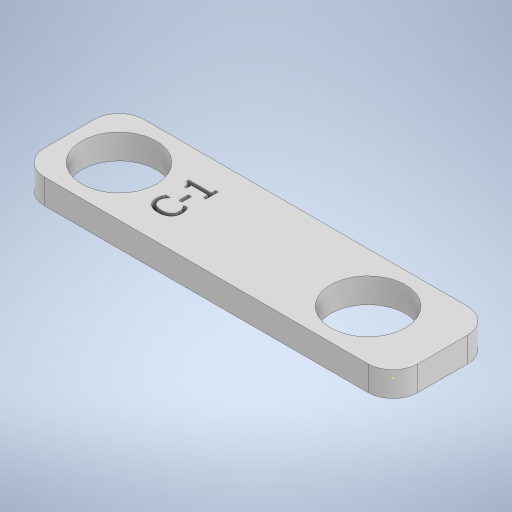
# Autodesk Inventor part: Parts_Combiner
Saved by Autodesk Inventor 2024.3 (Build 283343000, 343)
## iProperties
Created: 2024-08-06
Part Number: Parts_Combiner
Material: Generic
Document SubType Name: Modeling
Designer: lordk
Density: 1 g/cm^3
Appearance: Default
Author: lordk
Autodesk Inventor part; units mm, degrees
ref_plane "YZ Plane" through (0, 0, 0) normal (1, 0, 0) x (0, 1, 0)
ref_plane "XZ Plane" through (0, 0, 0) normal (0, 1, 0) x (-1, 0, 0)
ref_plane "XY Plane" through (0, 0, 0) normal (0, 0, 1) x (1, 0, 0)
sketch "Sketch1" plane through (0, 0, 0) normal (0, 1, 0) x (-1, 0, 0)
  line L0 (0, 0) -> (15, 0)
  line L1 (15, 0) -> (15, -4)
  line L2 (15, -4) -> (0, -4)
  line L3 (0, -4) -> (0, 0)
  dimension "d0" = 15
  dimension "d1" = 4
  constraints: 8 end point, 2 parallel, 1 horizontal, 1 perpendicular
  measures "d0" distance of L1.end L2.end
  measures "d1" distance of L0.end L1.end
extrude "Extrusion1" add sketch "Sketch1" along normal blind 1
sketch "Sketch2" plane through (0, 1, 0) normal (0, 1, 0) x (1, 0, 0)
  line L0 (0, 4) -> (-15, 4) projected
  line L1 (-15, 4) -> (-15, 0) projected
  point P0 (0, 0)
  point P1 (-13, 2)
  dimension "d18" = 2
  dimension "d19" = 2
  measures "d18" distance from line of L0 point (-13, 2)
  measures "d19" distance from line of L1 point (-13, 2)
hole "Hole1" at (-13, 1, -2) direction (0, -1, 0) diameter 3 depth 5 tip angle 118
sketch "Sketch3" plane through (0, 1, 0) normal (0, 1, 0) x (1, 0, 0)
  line L0 (0, 0) -> (0, 4) projected
  line L1 (0, 4) -> (-15, 4) projected
  point P0 (-3, 2)
  dimension "d20" = 3
  dimension "d21" = 2
  measures "d20" distance from line of L0 point (-3, 2)
  measures "d21" distance from line of L1 point (-3, 2)
hole "Hole2" at (-3, 1, -2) direction (0, -1, 0) diameter 3 depth 5 tip angle 118
sketch "Sketch4" plane through (0, 1, 0) normal (0, 1, 0) x (1, 0, 0)
  point P0 (0, 0)
fillet "Fillet1" radius 1 4 edges at (0, 0.5, 0) (0, 0.5, -4) (-15, 0.5, 0) (-15, 0.5, -4)
sketch "Sketch5" plane through (0, 1, 0) normal (0, 1, 0) x (1, 0, 0)
  line L0 (-11, 1) -> (-11, 3) construction
  line L1 (-11, 3) -> (-5, 3) construction
  line L2 (-5, 3) -> (-5, 1) construction
  line L3 (-5, 1) -> (-11, 1) construction
  line L4 (-1, 4) -> (-14, 4) projected
  line L5 (-14, 0) -> (-1, 0) projected
  line L6 (0, 1) -> (0, 3) projected
  line L7 (-15, 3) -> (-15, 1) projected
  spline S0 degree 2 poles (-9.9643, 1.4919) (-9.9643, 1.3947) (-10.03, 1.2301) (-10.0956, 1.1702) knots 0 0 0 1 2 2 2
  spline S1 degree 2 poles (-10.0956, 1.1702) (-10.1605, 1.1102) (-10.3549, 1.0446) (-10.4814, 1.0446) knots 0 0 0 1 2 2 2
  spline S2 degree 2 poles (-10.4814, 1.0446) (-10.607, 1.0446) (-10.7934, 1.1086) (-10.8622, 1.1694) knots 0 0 0 1 2 2 2
  spline S3 degree 2 poles (-10.8622, 1.1694) (-10.9295, 1.2293) (-11, 1.393) (-11, 1.4943) knots 0 0 0 1 2 2 2
  spline S4 degree 2 poles (-11, 1.4943) (-11, 1.5446) (-10.9854, 1.6329) (-10.9741, 1.6702) knots 0 0 0 1 2 2 2
  spline S5 degree 2 poles (-10.9741, 1.6702) (-10.9635, 1.7026) (-10.9335, 1.7699) (-10.9157, 1.8031) knots 0 0 0 1 2 2 2
  line L8 (-10.9157, 1.8031) -> (-10.7553, 1.8031)
  line L9 (-10.7553, 1.8031) -> (-10.7553, 1.7925)
  spline S6 degree 2 poles (-10.7553, 1.7925) (-10.7715, 1.7747) (-10.8169, 1.7196) (-10.8387, 1.6799) knots 0 0 0 1 2 2 2
  spline S7 degree 2 poles (-10.8387, 1.6799) (-10.8598, 1.6418) (-10.8865, 1.5519) (-10.8865, 1.4935) knots 0 0 0 1 2 2 2
  spline S8 degree 2 poles (-10.8865, 1.4935) (-10.8865, 1.4295) (-10.8339, 1.3152) (-10.7836, 1.2723) knots 0 0 0 1 2 2 2
  spline S9 degree 2 poles (-10.7836, 1.2723) (-10.7326, 1.2301) (-10.5778, 1.1831) (-10.4814, 1.1831) knots 0 0 0 1 2 2 2
  spline S10 degree 2 poles (-10.4814, 1.1831) (-10.3784, 1.1831) (-10.2301, 1.2326) (-10.1791, 1.2755) knots 0 0 0 1 2 2 2
  spline S11 degree 2 poles (-10.1791, 1.2755) (-10.1297, 1.3177) (-10.0794, 1.4303) (-10.0794, 1.4935) knots 0 0 0 1 2 2 2
  spline S12 degree 2 poles (-10.0794, 1.4935) (-10.0794, 1.5511) (-10.1078, 1.6491) (-10.1288, 1.6872) knots 0 0 0 1 2 2 2
  spline S13 degree 2 poles (-10.1288, 1.6872) (-10.1499, 1.7237) (-10.1937, 1.778) (-10.2091, 1.7934) knots 0 0 0 1 2 2 2
  line L10 (-10.2091, 1.7934) -> (-10.2091, 1.8031)
  line L11 (-10.2091, 1.8031) -> (-10.0502, 1.8031)
  spline S14 degree 2 poles (-10.0502, 1.8031) (-10.0348, 1.7699) (-10.0065, 1.7115) (-9.9935, 1.6702) knots 0 0 0 1 2 2 2
  spline S15 degree 2 poles (-9.9935, 1.6702) (-9.9789, 1.6264) (-9.9643, 1.5519) (-9.9643, 1.4919) knots 0 0 0 1 2 2 2
  line L12 (-10.359, 2.265) -> (-10.359, 1.8865)
  line L13 (-10.359, 1.8865) -> (-10.4806, 1.8865)
  line L14 (-10.4806, 1.8865) -> (-10.4806, 2.265)
  line L15 (-10.4806, 2.265) -> (-10.359, 2.265)
  line L16 (-9.9822, 2.9643) -> (-9.9822, 2.4765)
  line L17 (-9.9822, 2.4765) -> (-10.0843, 2.4765)
  line L18 (-10.0843, 2.4765) -> (-10.0843, 2.658)
  line L19 (-10.0843, 2.658) -> (-10.7545, 2.658)
  line L20 (-10.7545, 2.658) -> (-10.7545, 2.4765)
  line L21 (-10.7545, 2.4765) -> (-10.846, 2.4765)
  spline S16 degree 2 poles (-10.846, 2.4765) (-10.846, 2.5794) (-10.9044, 2.6767) (-10.9854, 2.6831) knots 0 0 0 1 2 2 2
  line L22 (-10.9854, 2.6831) -> (-10.9854, 2.7869)
  line L23 (-10.9854, 2.7869) -> (-10.0843, 2.7869)
  line L24 (-10.0843, 2.7869) -> (-10.0843, 2.9643)
  line L25 (-10.0843, 2.9643) -> (-9.9822, 2.9643)
  point P0 (0, 0)
  point P1 (-8, 1)
  dimension "d23" = 1
  dimension "d24" = 1
  dimension "d25" = 5
  dimension "d26" = 4
  constraints: 1 midpoint, 2 other
  measures "d23" distance between parallel lines of L4 L1
  measures "d24" distance from line of L5 point (-8, 1)
  measures "d25" distance between parallel lines of L6 L2
  measures "d26" distance between parallel lines of L7 L0
extrude "Extrusion2" cut sketch "Sketch5" against normal blind 0.5
body "Solid1"
